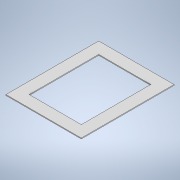
# Autodesk Inventor part: Plancha
Saved by Autodesk Inventor 2022.6 (Build 266554000, 554)
## iProperties
Created: 2025-01-14
Part Number: Plancha
Material: Genérico
Document SubType Name: Modeling
Designer: johan
Density: 1 g/cm^3
Appearance: Valor por defecto
Author: johan
Autodesk Inventor part; units mm, degrees
ref_plane "YZ Plane" through (0, 0, 0) normal (1, 0, 0) x (0, 1, 0)
ref_plane "XZ Plane" through (0, 0, 0) normal (0, 1, 0) x (-1, 0, 0)
ref_plane "XY Plane" through (0, 0, 0) normal (0, 0, 1) x (1, 0, 0)
sketch "Boceto1" plane through (0, 0, 0) normal (0, 1, 0) x (-1, 0, 0)
  line L0 (0, 0) -> (180, 0)
  line L1 (180, 0) -> (180, -240)
  line L2 (180, -240) -> (0, -240)
  line L3 (0, -240) -> (0, 0)
  line L4 (220, -280) -> (220, 40)
  line L5 (220, 40) -> (-40, 40)
  line L6 (-40, 40) -> (-40, -280)
  line L7 (-40, -280) -> (220, -280)
  dimension "d0" = 180
  dimension "d1" = 240
  dimension "d2" = 40
  constraints: 16 end point, 4 parallel, 2 perpendicular, 1 horizontal, 3 other
  measures "d0" distance of L1.end L2.end
  measures "d1" distance of L0.end L1.end
  measures "d2" distance between parallel lines of L1 L4
extrude "Extrusión1" add sketch "Boceto1" along normal blind 3
